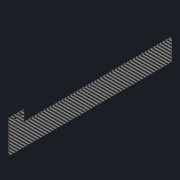
# Autodesk Inventor part: s_carbon_plate2
Saved by Autodesk Inventor 2022 (Build 260153000, 153)
## iProperties
Created: 2021-08-20
Part Number: s_carbon_plate2
Material: CFRP
Document SubType Name: Sheet Metal
Designer: yuta0
Density: 1.43 g/cm^3
Sheet Metal Rule: Default_mm
Appearance: カーボンファイバー
Author: yuta0
Autodesk Inventor part; units mm, degrees
ref_plane "YZ Plane" through (0, 0, 0) normal (1, 0, 0) x (0, 1, 0)
ref_plane "XZ Plane" through (0, 0, 0) normal (0, 1, 0) x (-1, 0, 0)
ref_plane "XY Plane" through (0, 0, 0) normal (0, 0, 1) x (1, 0, 0)
sketch "スケッチ1" plane through (0, 0, 0) normal (1, 0, 0) x (0, 1, 0)
  line L0 (-20.4, 102.5) -> (20.4, 102.5)
  line L1 (20.4, 102.5) -> (20.4, -102.5)
  line L2 (20.4, -102.5) -> (-20.4, -102.5)
  line L3 (-20.4, -102.5) -> (-20.4, 102.5)
  line L4 (-20.4, 102.5) -> (20.4, -102.5) construction
  line L5 (20.4, 102.5) -> (-20.4, -102.5) construction
  point P0 (0, 0)
  dimension "d0" = 40.8
  dimension "d1" = 205
  measures "d0" distance of L0.start L0.end
  measures "d1" distance of L0.end L1.end
extrude "プレート1" add sketch "スケッチ1" along normal mid plane 1
sketch "スケッチ2" plane through (0.5, 0, 0) normal (1, 0, 0) x (0, 0, -1)
  line L0 (-102.5, 20.4) -> (102.5, 20.4) projected
  line L1 (-102.5, -20.4) -> (-102.5, 20.4) projected
  point P0 (0, 0)
  point P1 (-95.5, 16.4)
  point P2 (-87.5, 16.4)
  dimension "d3" = 4
  dimension "d4" = 7
  dimension "d5" = 8
  constraints: 1 horizontal alignment
  measures "d3" distance from line of L0 point (-95.5, 16.4)
  measures "d4" distance from line of L1 point (-95.5, 16.4)
  measures "d5" distance of point (-95.5, 16.4) point (-87.5, 16.4)
hole "穴1" at (0.5, 16.4, 95.5) at (0.5, 16.4, 87.5) direction (-1, 0, 0) diameter 3.2 end through all clearance for "Socket Head Cap Screw" size "M3" standard "Ansi Metric M Profile"
sketch "スケッチ3" plane through (-0.5, 0, 0) normal (-1, 0, 0) x (0, 0, 1)
  line L0 (-102.5, 20.4) -> (-102.5, -20.4) projected
  line L1 (-102.5, 20.4) -> (83.5, 20.4)
  line L2 (83.5, 20.4) -> (83.5, 6.6)
  line L3 (83.5, 6.6) -> (-102.5, 6.6)
  line L4 (-102.5, 6.6) -> (-102.5, 20.4)
  line L5 (-102.5, -20.4) -> (102.5, -20.4) projected
  line L6 (102.5, -20.4) -> (102.5, 20.4) projected
  point P0 (0, 0)
  point P1 (-102.5, 6.6)
  dimension "d14" = 19
  dimension "d18" = 13.8
  constraints: 8 end point, 2 parallel, 1 horizontal, 1 perpendicular
  measures "d14" distance between parallel lines of L6 L2
  measures "d18" distance between parallel lines of L3 L1
extrude "押し出し1" cut sketch "スケッチ3" against normal blind 10
fillet "コーナーR1" radius 1 4 edges at (0, -20.4, 102.5) (0, -20.4, -102.5) (0, 6.6, -102.5) (0, 6.6, 83.5)
equation "\"d11\" = Thickness"
equation "\"d2\" = Thickness"
equation "\"BendRadius\" = Thickness"
equation "\"BendReliefWidth\" = Thickness"
equation "\"BendReliefDepth\" = 0.5 * Thickness"
equation "\"CornerReliefSize\" = 4 * Thickness"
equation "\"MinimumRemnant\" = 2 * Thickness"
equation "\"TransitionRadius\" = BendRadius"
equation "\"JacobiRadiusSize\" = BendRadius"
equation "\"GapSize\" = Thickness"
equation "\"Thickness\" = 1"
